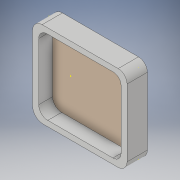
# Autodesk Inventor part: GoPro_Cap_Lens
Saved by Autodesk Inventor 2019 (Build 230136000, 136)
## iProperties
Created: 2019-02-06
Part Number: GoPro_Cap_Lens
Material: Generic
Document SubType Name: Modeling
Designer: jmc
Density: 1 g/cm^3
Appearance: Default
Author: jmc
Autodesk Inventor part; units mm, degrees
ref_plane "YZ Plane" through (0, 0, 0) normal (1, 0, 0) x (0, 1, 0)
ref_plane "XZ Plane" through (0, 0, 0) normal (0, 1, 0) x (-1, 0, 0)
ref_plane "XY Plane" through (0, 0, 0) normal (0, 0, 1) x (1, 0, 0)
sketch "Sketch1" plane through (-3.508, -14.003, 0) normal (0, 0, 1) x (1, 0, 0)
  line L0 (-3.495, 25.7995) -> (-3.495, 3.5141)
  line L1 (28.511, 26.087) -> (28.511, 3.1543)
  line L2 (0.0191, 0) -> (25.3567, 0)
  line L3 (25.4878, 29.006) -> (-0.274, 29.006)
  arc A0 (-3.495, 3.5141) -> (0.0191, 0) centre (0.0191, 3.5141) ccw
  arc A1 (25.3567, 0) -> (28.511, 3.1543) centre (25.3567, 3.1543) ccw
  arc A2 (28.511, 25.9828) -> (25.4878, 29.006) centre (25.4878, 25.9827) ccw
  arc A3 (-0.274, 29.006) -> (-3.495, 25.7995) centre (-0.2885, 25.7995) ccw
  line L4 (9.8544, 29.006) -> (9.8544, 34.006) construction
  point P0 (12.6069, 14.6206)
  dimension "d0" = 5
  constraints: 10 end point, 8 point on circle, 4 centre point, 2 point on line, 2 tangent, 1 vertical
  measures "d0" distance of L4.start L4.end
sketch "Sketch3" plane through (0, 0, 0) normal (0, 0, 1) x (1, 0, 0)
  arc A0 (-5.6755, 17.1176) -> (-9.37, 13.4398) centre (-5.6922, 13.4398) ccw
  line L0 (-9.37, 13.4398) -> (-9.37, -12.1215)
  arc A1 (-9.37, -12.1215) -> (-5.3393, -16.1522) centre (-5.3393, -12.1215) ccw
  line L1 (-5.3393, -16.1522) -> (23.723, -16.1522)
  arc A2 (23.723, -16.1522) -> (27.3409, -12.5343) centre (23.723, -12.5343) ccw
  line L2 (27.3409, 13.7696) -> (27.3409, -12.5343)
  arc A3 (27.3409, 13.65) -> (23.8733, 17.1176) centre (23.8733, 13.65) ccw
  line L3 (23.8733, 17.1176) -> (-5.6755, 17.1176)
  point P0 (0, 0)
  point P1 (25.003, 11.9798)
  point P2 (9.0989, 0.6176)
  constraints: 8 end point, 8 point on circle, 4 centre point, 1 point on line
extrude "Extrusion1" add sketch "Sketch3" along normal blind 7.886
shell "Shell1" thickness 2.5 removed faces 1 at (4.2862, 6.0277, 7.886)
ref_plane "Work Plane3" through (-5.6827, 14.6176, 2.5) normal (0, 0, 1) x (1, 0, 0)
sketch "Sketch4" plane through (-5.6827, 14.6176, 2.5) normal (0, 0, 1) x (1, 0, 0)
  point P0 (5.6827, -14.6176)
extrude "Extrusion2" cut sketch "Sketch1" along normal blind 21
sketch "Sketch5" plane through (-5.6827, 14.6176, 2.5) normal (0, 0, 1) x (1, 0, 0)
  arc A0 (0.3621, 0) -> (-1.1873, -1.9071) centre (1.8862, -2.8211) ccw projected
  line L0 (0.3621, 0) -> (0, 0) projected
  arc A1 (0, 0) -> (-1.1873, -1.1778) centre (-0.0094, -1.1778) ccw projected
  line L1 (-1.1873, -1.1778) -> (-1.1873, -1.9071) projected
  arc A2 (-1.1873, -26.0642) -> (0.6634, -28.2698) centre (2.1939, -25.1065) ccw projected
  line L2 (-1.1873, -26.0642) -> (-1.1873, -26.7391) projected
  arc A3 (-1.1873, -26.7391) -> (0.3435, -28.2698) centre (0.3435, -26.7391) ccw projected
  line L3 (0.3435, -28.2698) -> (0.6634, -28.2698) projected
  arc A4 (28.9771, -28.2698) -> (30.5236, -26.4645) centre (27.5315, -25.4663) ccw projected
  line L4 (28.9771, -28.2698) -> (29.4057, -28.2698) projected
  arc A5 (29.4057, -28.2698) -> (30.5236, -27.1519) centre (29.4057, -27.1519) ccw projected
  line L5 (30.5236, -27.1519) -> (30.5236, -26.4645) projected
  arc A6 (30.5236, -1.6612) -> (29.1395, 0) centre (27.6625, -2.6379) ccw projected
  line L6 (30.5236, -1.6612) -> (30.5236, -0.9676) projected
  arc A7 (30.5236, -0.9676) -> (29.556, 0) centre (29.556, -0.9676) ccw projected
  line L7 (29.556, 0) -> (29.1395, 0) projected
  point P0 (5.6827, -14.6176)
extrude "Extrusion3" add sketch "Sketch5" along normal up to surface (5.386 mm away)
sketch "Sketch6" plane through (-5.6827, 14.6176, 2.5) normal (0, 0, 1) x (1, 0, 0)
  arc A0 (27.5315, -28.6206) -> (30.6857, -25.4663) centre (27.5315, -25.4663) ccw projected
  line L0 (2.1939, -28.6206) -> (27.5315, -28.6206) projected
  arc A1 (-1.3203, -25.1065) -> (2.1939, -28.6206) centre (2.1939, -25.1065) ccw projected
  line L1 (-1.3203, -2.8211) -> (-1.3203, -25.1065) projected
  arc A2 (1.9007, 0.3854) -> (-1.3203, -2.8211) centre (1.8862, -2.8211) ccw projected
  line L2 (27.6625, 0.3854) -> (1.9007, 0.3854) projected
  arc A3 (30.6857, -2.6378) -> (27.6625, 0.3854) centre (27.6625, -2.6379) ccw projected
  line L3 (30.6857, -25.4663) -> (30.6857, -2.6378) projected
  point P0 (5.6827, -14.6176)
extrude "Extrusion4" add sketch "Sketch6" against normal up to surface (2.5 mm away)
body "Solid1"
